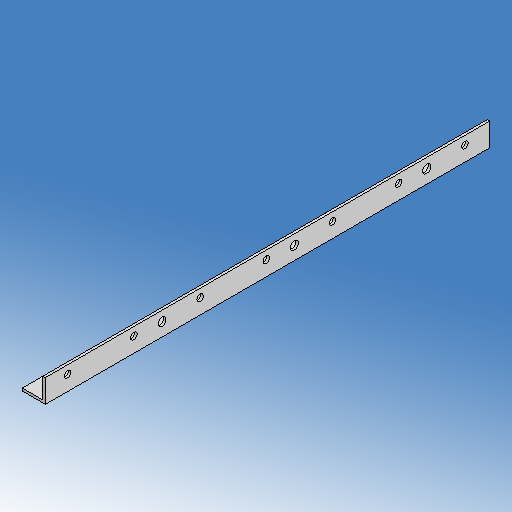
# Autodesk Inventor part: BatteryDrawer_AngleBrackets
Saved by Autodesk Inventor 2025 (Build 290162000, 162)
## iProperties
Created: 2024-08-04
Part Number: BatteryDrawer_AngleBrackets
Material: Generic
Document SubType Name: Modeling
Designer: seene
Density: 1 g/cm^3
Appearance: Default
Author: seene
Autodesk Inventor part; units mm, degrees
ref_plane "YZ Plane" through (0, 0, 0) normal (1, 0, 0) x (0, 1, 0)
ref_plane "XZ Plane" through (0, 0, 0) normal (0, 1, 0) x (-1, 0, 0)
ref_plane "XY Plane" through (0, 0, 0) normal (0, 0, 1) x (1, 0, 0)
sketch "Sketch1" plane through (0, 0, 0) normal (1, 0, 0) x (0, 1, 0)
  line L0 (0, 0) -> (203.2, 0) construction
  line L1 (203.2, 0) -> (203.2, 25.4) construction
  line L2 (203.2, 25.4) -> (0, 25.4) construction
  line L3 (0, 25.4) -> (0, 0) construction
  line L4 (0, 0) -> (25.4, 0) construction
  line L5 (25.4, 0) -> (25.4, -609.6) construction
  line L6 (25.4, -609.6) -> (0, -609.6) construction
  line L7 (0, -609.6) -> (0, 0) construction
  circle A0 centre (14.2875, -23.8125) radius 11.1125 construction
  line L8 (-1.5875, -12.7) -> (150.8125, -12.7) construction
  line L9 (114.3, -12.7) -> (25.4, -12.7) construction
  line L10 (25.4, -12.7) -> (25.4, -419.1) construction
  line L11 (25.4, -419.1) -> (114.3, -419.1) construction
  line L12 (114.3, -419.1) -> (114.3, -12.7) construction
  circle A1 centre (14.2875, -23.8125) radius 7.9375 construction
  circle A2 centre (14.2875, -23.8125) radius 3.175
  circle A3 centre (12.7, -114.3) radius 3.9688
  circle A4 centre (12.7, -241.3) radius 3.9688
  circle A5 centre (12.7, -368.3) radius 3.9688
  circle A6 centre (12.7, -495.3) radius 3.9688 construction
  circle A7 centre (14.2875, -87.3125) radius 3.175
  circle A8 centre (14.2875, -87.3125) radius 11.1125 construction
  circle A9 centre (14.2875, -150.8125) radius 3.175
  circle A10 centre (14.2875, -150.8125) radius 11.1125 construction
  circle A11 centre (14.2875, -214.3125) radius 3.175
  circle A12 centre (14.2875, -214.3125) radius 11.1125 construction
  circle A13 centre (14.2875, -277.8125) radius 3.175
  circle A14 centre (14.2875, -277.8125) radius 11.1125 construction
  circle A15 centre (14.2875, -341.3125) radius 3.175
  circle A16 centre (14.2875, -341.3125) radius 11.1125 construction
  circle A17 centre (14.2875, -404.8125) radius 3.175
  circle A18 centre (14.2875, -404.8125) radius 11.1125 construction
  line L13 (0, -2.4888) -> (22.225, -2.4888)
  line L14 (22.225, -2.4888) -> (22.225, -428.625)
  line L15 (22.225, -428.625) -> (0, -428.625)
  line L16 (0, -428.625) -> (0, -2.4888)
  dimension "d0" = 203.2
  dimension "d1" = 25.4
  dimension "d2" = 25.4
  dimension "d3" = 609.6
  dimension "d4" = 12.7
  dimension "d6" = 22.225
  dimension "d7" = 406.4
  dimension "d8" = 88.9
  dimension "d10" = 15.875
  dimension "d11" = 6.35
  dimension "d12" = 7.9375
  dimension "d13" = 12.7
  dimension "d14" = 114.3
  dimension "d17" = 127
  dimension "d24" = 63.5
  dimension "d29" = 22.225
  constraints: 34 end point, 19 centre point, 9 coincident, 8 parallel, 5 horizontal, 4 perpendicular, 3 tangent, 2 vertical, 1 collinear, 1 point on line, 30 other
  measures "d0" distance of L2.end L1.end
  measures "d1" distance of L1.end L0.end
  measures "d2" distance of L5.end L6.end
  measures "d3" distance of L4.end L5.end
  measures "d4" distance between parallel lines of L8 L0
  measures "d6" diameter of A0
  measures "d7" distance of L11.end L9.start
  measures "d8" distance of L10.end L11.end
  measures "d10" diameter of A1
  measures "d11" diameter of A2
  measures "d12" diameter of A3
  measures "d13" distance from line of L7 A3.centre
  measures "d14" distance from line of A3.centre L0
  measures "d17" distance of A3.centre A4.centre
  measures "d24" distance of A2.centre A7.centre
  measures "d29" distance of L14.end L15.end
extrude "Extrusion1" add sketch "Sketch1" along normal blind 2.3876
sketch "Sketch2" plane through (0, 0, -2.4888) normal (0, 0, 1) x (1, 0, 0)
  line L0 (0, 0) -> (-19.8374, 0)
  line L1 (-19.8374, 0) -> (-19.8374, 2.3876)
  line L2 (-19.8374, 2.3876) -> (0, 2.3876)
  line L3 (0, 2.3876) -> (0, 0)
  dimension "d32" = 19.8374
  dimension "d33" = 2.3876
  constraints: 8 end point, 2 parallel, 1 horizontal, 1 perpendicular
  measures "d32" distance of L1.end L2.end
  measures "d33" distance of L0.end L1.end
extrude "Extrusion2" add sketch "Sketch2" against normal up to surface (426.1362 mm away)
sketch "Sketch3" plane through (-19.8374, 2.3876, -2.4888) normal (0, 1, 0) x (1, 0, 0)
  circle A0 centre (9.9187, 25.4) radius 3.175
  line L0 (19.8374, 0) -> (0, 0) projected
  line L1 (9.9187, 0) -> (9.9187, 25.4) construction
  circle A1 centre (9.9187, 400.7362) radius 3.175
  line L2 (19.8374, 426.1362) -> (0, 426.1362) construction
  point P0 (19.8374, -2.4888)
  dimension "d36" = 6.35
  dimension "d37" = 25.4
  dimension "d38" = 6.35
  dimension "d39" = 25.4
  constraints: 2 centre point, 2 end point, 1 midpoint, 1 vertical, 1 vertical alignment
  measures "d36" diameter of A0
  measures "d37" distance from line of L1.end L0
  measures "d38" diameter of A1
  measures "d39" distance from line of L2 A1.centre
extrude "Extrusion3" cut sketch "Sketch3" against normal through all
body "Solid1"
